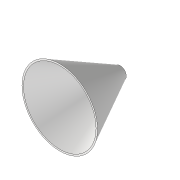
# Autodesk Inventor part: Speicher_1
Saved by Autodesk Inventor 2020 (Build 240168000, 168)
## iProperties
Created: 2020-04-19
Part Number: Speicher_1
Material: Generisch
Document SubType Name: Modeling
Designer: franz
Density: 1 g/cm^3
Appearance: Vorgabe
Author: franz
Autodesk Inventor part; units mm, degrees
ref_plane "YZ Plane" through (0, 0, 0) normal (1, 0, 0) x (0, 1, 0)
ref_plane "XZ Plane" through (0, 0, 0) normal (0, 1, 0) x (-1, 0, 0)
ref_plane "XY Plane" through (0, 0, 0) normal (0, 0, 1) x (1, 0, 0)
sketch "Skizze2" plane through (0, 0, 0) normal (0, 1, 0) x (-1, 0, 0)
  line L0 (0, 68.6607) -> (0, -20.1415)
  line L1 (-5, 0) -> (-10, 0)
  line L2 (-10, 0) -> (-62.5, 100)
  line L3 (-62.5, 100) -> (-60, 100)
  line L4 (-60, 100) -> (-7.5, 0)
  line L5 (0, -44.1698) -> (0, 124.0283) projected
  point P0 (0, 0)
  dimension "d2" = 15
  dimension "d3" = 20
  dimension "d4" = 100
  dimension "d5" = 120
  constraints: 10 end point, 2 parallel, 1 collinear, 1 horizontal, 1 midpoint, 1 vertical
  measures "d2" diameter of L4.end L0
  measures "d3" diameter of L1.end L0
  measures "d4" distance between parallel lines of L1 L3
  measures "d5" diameter of L3.end L0
revolve "Umdrehung1" add sketch "Skizze2" angle 360 about axis through (0, 0, 68.6607) along (0, 0, -1)
